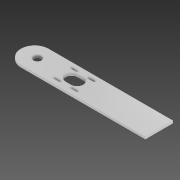
# Autodesk Inventor part: bovenarm - rechts
Saved by Autodesk Inventor 2020 (Build 240168000, 168)
## iProperties
Created: 2020-05-18
Part Number: bovenarm - rechts
Material: Generic
Document SubType Name: Modeling
Designer: stefa
Density: 1 g/cm^3
Appearance: Aluminum - Polished
Author: stefa
Autodesk Inventor part; units mm, degrees
ref_plane "YZ Plane" through (0, 0, 0) normal (1, 0, 0) x (0, 1, 0)
ref_plane "XZ Plane" through (0, 0, 0) normal (0, 1, 0) x (-1, 0, 0)
ref_plane "XY Plane" through (0, 0, 0) normal (0, 0, 1) x (1, 0, 0)
sketch "Sketch1" plane through (0, 0, 0) normal (0, 1, 0) x (-1, 0, 0)
  line L0 (0, 0) -> (250, 0)
  line L1 (250, 0) -> (250, -50)
  line L2 (250, -50) -> (0, -50)
  line L3 (0, -50) -> (0, 0)
  circle A0 centre (220, -25) radius 7
  line L4 (158.262, -25) -> (148.262, -25) construction
  line L5 (158.262, -13.9) -> (148.262, -13.9)
  line L6 (148.262, -36.1) -> (158.262, -36.1)
  arc A1 (158.262, -36.1) -> (158.262, -13.9) centre (158.262, -25) ccw
  arc A2 (148.262, -13.9) -> (148.262, -36.1) centre (148.262, -25) ccw
  line L7 (173.762, -40.5) -> (163.762, -40.5) construction
  line L8 (173.762, -38.95) -> (163.762, -38.95)
  line L9 (163.762, -42.05) -> (173.762, -42.05)
  arc A3 (173.762, -42.05) -> (173.762, -38.95) centre (173.762, -40.5) ccw
  arc A4 (163.762, -38.95) -> (163.762, -42.05) centre (163.762, -40.5) ccw
  line L10 (132.762, -42.05) -> (142.762, -42.05)
  arc A5 (142.762, -42.05) -> (142.762, -38.95) centre (142.762, -40.5) ccw
  line L11 (142.762, -40.5) -> (132.762, -40.5) construction
  line L12 (142.762, -38.95) -> (132.762, -38.95)
  arc A6 (132.762, -38.95) -> (132.762, -42.05) centre (132.762, -40.5) ccw
  line L13 (163.762, -11.05) -> (173.762, -11.05)
  arc A7 (173.762, -11.05) -> (173.762, -7.95) centre (173.762, -9.5) ccw
  line L14 (173.762, -9.5) -> (163.762, -9.5) construction
  line L15 (173.762, -7.95) -> (163.762, -7.95)
  arc A8 (163.762, -7.95) -> (163.762, -11.05) centre (163.762, -9.5) ccw
  line L16 (132.762, -11.05) -> (142.762, -11.05)
  arc A9 (142.762, -11.05) -> (142.762, -7.95) centre (142.762, -9.5) ccw
  line L17 (142.762, -9.5) -> (132.762, -9.5) construction
  line L18 (142.762, -7.95) -> (132.762, -7.95)
  arc A10 (132.762, -7.95) -> (132.762, -11.05) centre (132.762, -9.5) ccw
  point P0 (153.262, -25)
  point P1 (168.762, -40.5)
  point P2 (137.762, -40.5)
  point P3 (168.762, -9.5)
  point P4 (137.762, -9.5)
  dimension "d0" = 250
  dimension "d1" = 50
  dimension "d16" = 14
  dimension "d18" = 25
  dimension "d24" = 22.2
  dimension "d25" = 3.1
  dimension "d26" = 10
  dimension "d27" = 10
  dimension "d28" = 66.738
  dimension "d29" = 25
  dimension "d30" = 30
  dimension "d31" = 15.5
  dimension "d32" = 15.5
  dimension "d35" = 31
  dimension "d38" = 31
  constraints: 48 end point, 20 point on circle, 11 centre point, 8 tangent, 5 parallel, 3 horizontal, 2 midpoint, 1 perpendicular, 1 vertical, 36 other
  measures "d0" distance of L1.end L2.end
  measures "d1" distance of L0.end L1.end
  measures "d16" diameter of A0
  measures "d18" distance from line of L0 A0.centre
  measures "d24" diameter of A2
  measures "d25" diameter of A4
  measures "d26" distance of L9.start L9.end
  measures "d27" distance of L6.start L6.end
  measures "d28" distance of A0.centre point (153.262, -25)
  measures "d29" distance from line of L0 point (153.262, -25)
  measures "d30" distance from line of L1 A0.centre
  measures "d31" horizontal distance of point (153.262, -25) point (168.762, -40.5)
  measures "d32" horizontal distance of point (168.762, -40.5) point (153.262, -25)
  measures "d35" distance of L9.start L10.start
  measures "d38" distance of L9.start L13.start
extrude "Extrusion1" add sketch "Sketch1" along normal blind 4
fillet "Fillet1" radius 25 2 edges at (-250, 2, 0) (-250, 2, -50)
equation "\"d18\" = 0.5 * d1"
body "Solid1"
